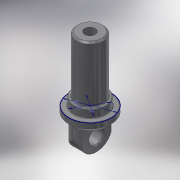
# Autodesk Inventor part: Base
Saved by Autodesk Inventor 2014 (Build 180170000, 170)
## iProperties
Created: 2013-09-01
Part Number: Base
Material: Steel
Document SubType Name: Modeling
Designer: Arto
Density: 7.85 g/cm^3
Appearance: Anodisé - Gris clair
Author: Arto
Autodesk Inventor part; units mm, degrees
ref_plane "YZ Plane" through (0, 0, 0) normal (1, 0, 0) x (0, 1, 0)
ref_plane "XZ Plane" through (0, 0, 0) normal (0, 1, 0) x (-1, 0, 0)
ref_plane "XY Plane" through (0, 0, 0) normal (0, 0, 1) x (1, 0, 0)
sketch "Sketch1" plane through (0, 0, 0) normal (0, 0, 1) x (1, 0, 0)
  circle A0 centre (0, 0) radius 40
  circle A1 centre (0, 0) radius 30
  circle A2 centre (0, 0) radius 25
  dimension "d0" = 80
  dimension "d1" = 60
  dimension "d6" = 50
  constraints: 3 centre point, 3 coincident
  measures "d0" diameter of A0
  measures "d1" diameter of A1
  measures "d6" diameter of A2
extrude "Extrusion1" add sketch "Sketch1" against normal blind 20 contours A0 | A1 | A2
extrude "Extrusion2" add sketch "Sketch1" along normal blind 15 contours A1 | A2
extrude "Extrusion3" add sketch "Sketch1" along normal blind 120 contours A2
chamfer "Chamfer1" distance 10 angle 45 1 edges at (-40, 0, -20)
chamfer "Chamfer2" distance 1 angle 45 4 edges at (-40, 0, 0) (-30, 0, 15) (-30, 0, 0) (-25, 0, 15)
sketch "Sketch2" plane through (0, 0, -20) normal (0, 0, -1) x (-1, 0, 0)
  circle A0 centre (0, 0) radius 30 projected
  line L0 (-12.5, 27.2718) -> (-12.5, -27.2718)
  line L1 (12.5, 27.2718) -> (12.5, -27.2718)
  dimension "d15" = 25
  constraints: 4 end point, 4 point on circle, 2 parallel, 1 vertical
  measures "d15" distance between parallel lines of L1 L0
extrude "Extrusion4" add sketch "Sketch2" along normal blind 50 contours L1 A0 L0
sketch "Sketch3" plane through (12.5, -27.2718, -20) normal (1, 0, 0) x (0, 0, -1)
  line L0 (50, 54.5436) -> (50, 57.2718) construction
  line L1 (50, -2.7282) -> (50, 0) construction
  arc A0 (20, -2.7282) -> (20, 57.2718) centre (20, 27.2718) ccw
  line L2 (20, 57.2718) -> (20, -2.7282) construction
  line L3 (20, 57.2718) -> (80, 57.2718) construction
  line L4 (20, 57.2718) -> (55.8157, 57.2718)
  line L5 (20, -2.7282) -> (55.8157, -2.7282)
  line L6 (50, 54.5436) -> (50, 0) construction
  line L7 (55.8157, -2.7282) -> (55.8157, 57.2718)
  point P0 (-20, 27.2718)
  dimension "d19" = 90
  dimension "d48" = 30
  constraints: 10 end point, 3 point on line, 2 midpoint, 2 parallel, 2 point on circle, 1 centre point, 1 horizontal, 1 perpendicular, 1 tangent
  measures "d19" angle of L2 L3
  measures "d48" radius of A0
extrude "Extrusion5" cut sketch "Sketch3" against normal through all
hole "Hole1" at (12.5, 0, -45) direction (-1, 0, 0) diameter 26 end through all
chamfer "Chamfer3" distance 2 angle 45 2 edges at (12.5, 0, -20) (-12.5, 0, -20)
hole "Hole2" at (0, 0, 120) direction (0, 0, -1) diameter 20 depth 120
chamfer "Chamfer4" distance 3 angle 45 1 edges at (-25, 0, 120)
chamfer "Chamfer5" distance 1 angle 45 2 edges at (-12.5, 0, -70) (12.5, 0, -70)
chamfer "Chamfer6" distance 2 angle 45 2 edges at (12.5, 0, -32) (-12.5, 0, -32)
body "Solid1"
